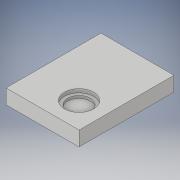
# Autodesk Inventor part: Saber plaque
Saved by Autodesk Inventor 2017 SP1 (Build 210196100, 196)
## iProperties
Created: 2017-11-06
Part Number: Saber plaque
Material: Generic
Document SubType Name: Modeling
Designer: rmainhar
Density: 1 g/cm^3
Appearance: Default
Author: rmainhar
Autodesk Inventor part; units mm, degrees
ref_plane "YZ Plane" through (0, 0, 0) normal (1, 0, 0) x (0, 1, 0)
ref_plane "XZ Plane" through (0, 0, 0) normal (0, 1, 0) x (-1, 0, 0)
ref_plane "XY Plane" through (0, 0, 0) normal (0, 0, 1) x (1, 0, 0)
sketch "Sketch1" plane through (0, 0, 0) normal (0, 1, 0) x (-1, 0, 0)
  line L0 (0, 0) -> (-127, 0)
  line L1 (-127, 0) -> (-127, -165.1)
  line L2 (-127, -165.1) -> (0, -165.1)
  line L3 (0, -165.1) -> (0, 0)
  dimension "d0" = 127
  dimension "d1" = 165.1
  constraints: 8 end point, 2 parallel, 1 horizontal, 1 perpendicular
  measures "d0" distance of L2.end L1.end
  measures "d1" distance of L1.end L0.end
extrude "Extrusion1" add sketch "Sketch1" along normal blind 25.4
sketch "Sketch2" plane through (0, 25.4, 0) normal (0, 1, 0) x (1, 0, 0)
  circle A0 centre (82.55, 44.45) radius 25.4
  line L0 (0, 0) -> (127, 0) projected
  line L1 (127, 0) -> (127, 165.1) projected
  line L2 (127, 165.1) -> (0, 165.1) projected
  line L3 (0, 165.1) -> (0, 0) projected
  dimension "d4" = 50.8
  dimension "d5" = 44.45
  dimension "d6" = 44.45
  constraints: 1 centre point
  measures "d4" diameter of A0
  measures "d5" horizontal distance of A0.centre L0.end
  measures "d6" distance from line of L0 A0.centre
extrude "Extrusion2" cut sketch "Sketch2" against normal blind 6.35 contours A0
sketch "Sketch3" plane through (82.55, 19.05, -44.45) normal (0, 1, 0) x (1, 0, 0)
  circle A0 centre (0, 0) radius 19.812
  point P0 (-82.55, -44.45)
  dimension "d9" = 39.624
  constraints: 1 centre point
  measures "d9" diameter of A0
extrude "Extrusion3" cut sketch "Sketch3" against normal blind 4.445
equation "\"d5\" = d6"
body "Solid1"
